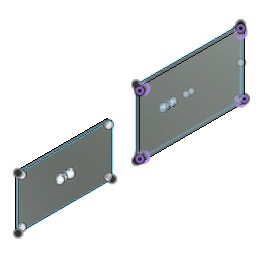
measurement_device(autodesk_model) (Autodesk Fusion 360 archive; units mm, degrees)
design "hakari"
Autodesk Fusion 360 part; units mm, degrees
sketch "スケッチ1" plane through (0, 0, 0) normal (1, 0, 0) x (0, 1, 0)
  line L0 (-45, 25) -> (95, 25)
  line L1 (100, 20) -> (100, -65)
  line L2 (95, -70) -> (-45, -70)
  line L3 (-50, -65) -> (-50, 20)
  arc A0 (-45, 25) -> (-50, 20) centre (-45, 20) ccw
  arc A1 (-50, -65) -> (-45, -70) centre (-45, -65) ccw
  arc A2 (100, 20) -> (95, 25) centre (95, 20) ccw
  arc A3 (95, -70) -> (100, -65) centre (95, -65) ccw
  line L4 (100, -70) -> (100, -22.5)
  circle A4 centre (28.7, -22.5) radius 1.5
  circle A5 centre (21.3, -22.5) radius 1.5
  circle A6 centre (-0.7, -22.5) radius 1.6
  circle A7 centre (-8.1, -22.5) radius 1.6
  line L5 (-12, -27) -> (3, -27)
  line L6 (6, -24) -> (6, -21)
  line L7 (3, -18) -> (-12, -18)
  line L8 (-15, -21) -> (-15, -24)
  arc A8 (-15, -24) -> (-12, -27) centre (-12, -24) ccw
  arc A9 (3, -27) -> (6, -24) centre (3, -24) ccw
  arc A10 (6, -21) -> (3, -18) centre (3, -21) ccw
  arc A11 (-12, -18) -> (-15, -21) centre (-12, -21) ccw
  point P0 (-50, 25)
  point P1 (100, 25)
  point P2 (-50, -70)
  dimension "d1" = 150
  dimension "d2" = 95
  dimension "d9" = 5
  dimension "d10" = 5
  dimension "d11" = 5
  dimension "d12" = 5
  dimension "d25" = 47.5
  dimension "d31" = 3
  dimension "d32" = 7.4
  dimension "d33" = 3
  dimension "d34" = 22
  dimension "d36" = 7.4
  dimension "d37" = 3.2
  dimension "d43" = 3.2
  dimension "d48" = 3
  dimension "d49" = 3
  dimension "d50" = 3
  dimension "d51" = 3
  constraint horizontal L0
  constraint vertical L1
  constraint horizontal L2
  constraint vertical L3
  constraint coincident P0 L0
  constraint coincident P0 L3
  constraint tangent L0 A0
  constraint tangent L3 A0
  constraint coincident P2 L2
  constraint coincident P2 L3
  constraint tangent L2 A1
  constraint tangent L3 A1
  constraint coincident P1 L0
  constraint coincident P1 L1
  constraint tangent L0 A2
  constraint tangent L1 A2
  constraint tangent L1 A3
  constraint tangent L2 A3
  constraint parallel L1 L4
  constraint horizontal L5
  constraint vertical L6
  constraint horizontal L7
  constraint vertical L8
  constraint tangent L5 A8
  constraint tangent L8 A8
  constraint tangent L5 A9
  constraint tangent L6 A9
  constraint tangent L6 A10
  constraint tangent L7 A10
  constraint tangent L7 A11
  constraint tangent L8 A11
  measures "d1" distance of P0 P1
  measures "d2" distance of P0 P2
  measures "d9" radius of A0
  measures "d10" radius of A1
  measures "d11" radius of A2
  measures "d12" radius of A3
  measures "d25" distance of L4.start L4.end
  measures "d31" diameter of A4
  measures "d32" distance of A4.centre A5.centre
  measures "d33" diameter of A5
  measures "d34" distance of A5.centre A6.centre
  measures "d36" distance of A6.centre A7.centre
  measures "d37" diameter of A7
  measures "d43" diameter of A6
  measures "d48" radius of A8
  measures "d49" radius of A9
  measures "d50" radius of A10
  measures "d51" radius of A11
extrude "押し出し1" add sketch "スケッチ1" along normal blind 5 contours L0 L1 L2 L3 A0 A1 A2 A3 L4 | A4 | A5 | A6 | A7 | L5 L6 L7 L8 A8 A9 A10 A11 makes body 1
sketch "スケッチ2" plane through (5, 0, 0) normal (1, 0, 0) x (0, 1, 0)
  line L0 (-45, -70) -> (95, -70)
  line L1 (100, -65) -> (100, 20)
  line L2 (95, 25) -> (-45, 25)
  line L3 (-50, 20) -> (-50, -65)
  line L4 (-220, -70) -> (-95, -70)
  line L5 (-90, -65) -> (-90, 0)
  line L6 (-95, 5) -> (-220, 5)
  line L7 (-225, 0) -> (-225, -65)
  arc A0 (-50, -65) -> (-45, -70) centre (-45, -65) ccw
  arc A1 (95, -70) -> (100, -65) centre (95, -65) ccw
  arc A2 (100, 20) -> (95, 25) centre (95, 20) ccw
  arc A3 (-45, 25) -> (-50, 20) centre (-45, 20) ccw
  arc A4 (-90, 0) -> (-95, 5) centre (-95, 0) ccw
  arc A5 (-220, 5) -> (-225, 0) centre (-220, 0) ccw
  arc A6 (-95, -70) -> (-90, -65) centre (-95, -65) ccw
  arc A7 (-225, -65) -> (-220, -70) centre (-220, -65) ccw
  circle A8 centre (-153.8, -32.5) radius 1.6
  circle A9 centre (-161.2, -32.5) radius 1.6
  line L8 (-165, -37) -> (-150, -37)
  line L9 (-147, -34) -> (-147, -31)
  line L10 (-150, -28) -> (-165, -28)
  line L11 (-168, -31) -> (-168, -34)
  arc A10 (-147, -31) -> (-150, -28) centre (-150, -31) ccw
  arc A11 (-165, -28) -> (-168, -31) centre (-165, -31) ccw
  arc A12 (-168, -34) -> (-165, -37) centre (-165, -34) ccw
  arc A13 (-150, -37) -> (-147, -34) centre (-150, -34) ccw
  point P0 (-225, -70)
  point P1 (-90, -70)
  point P2 (-225, 5)
  dimension "d5" = 135
  dimension "d6" = 75
  dimension "d13" = 5
  dimension "d14" = 5
  dimension "d15" = 5
  dimension "d16" = 5
  dimension "d19" = 3.2
  dimension "d20" = 3.2
  dimension "d54" = 3
  dimension "d55" = 3
  dimension "d56" = 3
  dimension "d57" = 3
  constraint horizontal L4
  constraint vertical L5
  constraint horizontal L6
  constraint vertical L7
  constraint tangent L5 A4
  constraint tangent L6 A4
  constraint coincident P2 L6
  constraint coincident P2 L7
  constraint tangent L6 A5
  constraint tangent L7 A5
  constraint coincident P1 L4
  constraint coincident P1 L5
  constraint tangent L4 A6
  constraint tangent L5 A6
  constraint coincident P0 L4
  constraint coincident P0 L7
  constraint tangent L4 A7
  constraint tangent L7 A7
  constraint horizontal L8
  constraint vertical L9
  constraint horizontal L10
  constraint vertical L11
  constraint tangent L9 A10
  constraint tangent L10 A10
  constraint tangent L10 A11
  constraint tangent L11 A11
  constraint tangent L8 A12
  constraint tangent L11 A12
  constraint tangent L8 A13
  constraint tangent L9 A13
  measures "d5" distance of P0 P1
  measures "d6" distance of P0 P2
  measures "d13" radius of A4
  measures "d14" radius of A5
  measures "d15" radius of A6
  measures "d16" radius of A7
  measures "d19" diameter of A8
  measures "d20" diameter of A9
  measures "d54" radius of A10
  measures "d55" radius of A11
  measures "d56" radius of A12
  measures "d57" radius of A13
extrude "押し出し5" cut sketch "スケッチ1" along normal blind 8 contours A7 bodies 1
extrude "押し出し6" cut sketch "スケッチ1" along normal blind 18 contours A6 bodies 1
extrude "押し出し7" add sketch "スケッチ2" against normal blind 4 separate body contours L4 L5 L6 L7 A4 A5 A6 A7 | L8 L9 L10 L11 A10 A11 A12 A13 makes body 2
extrude "押し出し8" add sketch "スケッチ1" against normal blind 4 contours L5 L6 L7 L8 A8 A9 A10 A11 bodies 1
extrude "押し出し9" add sketch "スケッチ2" against normal blind 8 contours L8 L9 L10 L11 A10 A11 A12 A13 bodies 2
copy_body "ボディ -> コンポーネント1" bodies 1 removing the originals makes body 3 in component "Component"
copy_body "ボディ -> コンポーネント2" bodies 2 removing the originals makes body 4 in component "Component'"
extrude "押し出し2" [rolled back] along distance -4 taper angle 0
extrude "押し出し3" [rolled back] along distance -8 taper angle 0
extrude "押し出し4" [rolled back] along distance -8 taper angle 0
component "Component" placed x (1, 0, 0) y (0, 1, 0) z (0, 0, 1) at (0, 0, 0)
component "Component'" placed x (1, 0, 0) y (0, 1, 0) z (0, 0, 1) at (0, 0, 0)
